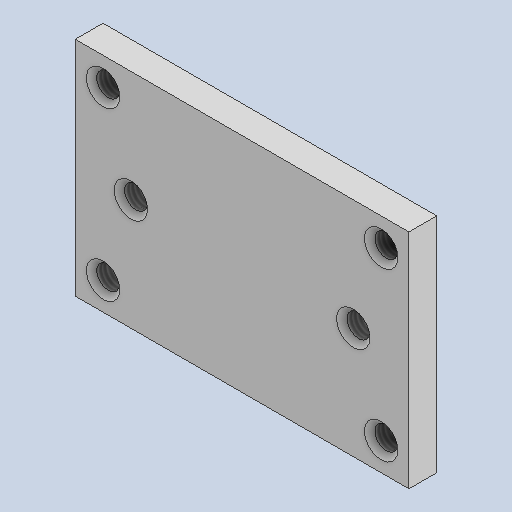
# Autodesk Inventor part: podstawka
Saved by Autodesk Inventor 2025.2 (Build 292293000, 293)
## iProperties
Created: 2026-05-07
Part Number: podstawka
Material: Ogólny
Document SubType Name: Modeling
Designer: muszy
Density: 1 g/cm^3
Appearance: Domyślna
Author: muszy
Autodesk Inventor part; units mm, degrees
ref_plane "YZ Plane" through (0, 0, 0) normal (1, 0, 0) x (0, 1, 0)
ref_plane "XZ Plane" through (0, 0, 0) normal (0, 1, 0) x (-1, 0, 0)
ref_plane "XY Plane" through (0, 0, 0) normal (0, 0, 1) x (1, 0, 0)
sketch "Szkic1" plane through (0, 0, 0) normal (0, 0, 1) x (1, 0, 0)
  line L0 (21.4781, -20) -> (21.4781, 20)
  line L1 (-21.5797, -20) -> (21.4781, -20)
  line L2 (-38.5219, 20) -> (-38.5219, -20)
  line L3 (-38.5219, -20) -> (-25.4723, -20)
  line L4 (-25.4723, -20) -> (-21.5797, -20)
  line L5 (-31.9971, 20) -> (-38.5219, 20)
  line L6 (21.4781, 20) -> (6.0004, 20)
  line L7 (6.0004, 20) -> (-31.9971, 20)
  point P0 (0, 0)
extrude "Wyciągnięcie proste1" add sketch "Szkic1" along normal blind 5
sketch "Szkic2" plane through (0, 0, 5) normal (0, 0, 1) x (1, 0, 0)
  circle A0 centre (16.4781, 15) radius 2.067 projected
  circle A1 centre (16.4781, -15) radius 2.067 projected
  circle A2 centre (-33.5219, -15) radius 2.067 projected
  circle A3 centre (-33.5219, 15) radius 2.067 projected
  point P0 (0, 0)
hole "Otwór1" at (16.4781, -15, 5) at (-33.5219, -15, 5) at (16.4781, 15, 5) at (-33.5219, 15, 5) direction (0, 0, -1) diameter 4.134 end through all countersink diameter 6 countersink angle 90 thread size "M5x0.8" class "6H" standard "ISO Metric profile"
sketch "Szkic3" plane through (0, 0, 5) normal (0, 0, 1) x (1, 0, 0)
  line L0 (21.4781, 20) -> (-38.5219, 20) projected
  line L1 (21.4781, -20) -> (21.4781, 20) projected
  line L2 (-38.5219, 20) -> (-38.5219, -20) projected
  point P0 (0, 0)
  point P1 (11.4781, 0)
  point P2 (-28.5219, 0)
  dimension "d9" = 20
  dimension "d10" = 10
  dimension "d11" = 20
  dimension "d12" = 10
  measures "d9" distance from line of L0 point (11.478, 0)
  measures "d10" distance from line of L1 point (11.478, 0)
  measures "d11" distance from line of L0 point (-28.522, 0)
  measures "d12" distance from line of L2 point (-28.522, 0)
hole "Otwór2" at (11.4781, 0, 5) at (-28.5219, 0, 5) direction (0, 0, -1) diameter 4.134 end through all countersink diameter 6 countersink angle 90 thread size "M5x0.8" class "6H" standard "ISO Metric profile"
